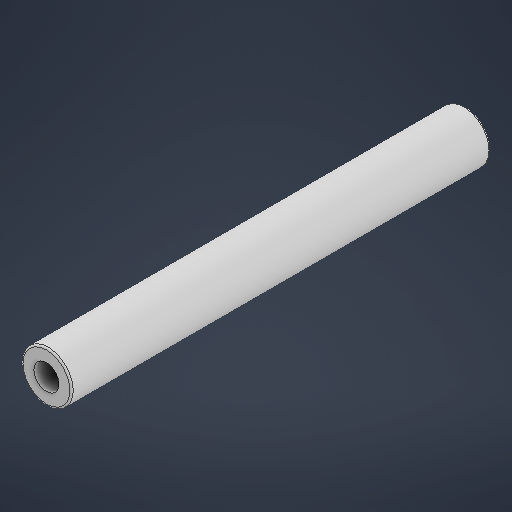
# Autodesk Inventor part: suport_bars
Saved by Autodesk Inventor 2025.3 (Build 293356000, 356)
## iProperties
Created: 2025-04-06
Part Number: suport_bars
Material: Generic
Document SubType Name: Modeling
Designer: Tiago
Density: 1 g/cm^3
Appearance: Default
Author: Tiago
Autodesk Inventor part; units mm, degrees
ref_plane "YZ Plane" through (0, 0, 0) normal (1, 0, 0) x (0, 1, 0)
ref_plane "XZ Plane" through (0, 0, 0) normal (0, 1, 0) x (-1, 0, 0)
ref_plane "XY Plane" through (0, 0, 0) normal (0, 0, 1) x (1, 0, 0)
sketch "Sketch1" plane through (0, 0, 0) normal (0, 0, 1) x (1, 0, 0)
  circle A0 centre (0, 0) radius 1.5
  circle A1 centre (0, 0) radius 3
  dimension "M3" = 3
  dimension "D" = 6
  constraints: 2 centre point, 2 coincident
  measures "M3" diameter of A0
  measures "D" diameter of A1
extrude "Extrusion3" add sketch "Sketch1" along normal blind 50
fillet "Fillet2" radius 0.2 2 edges at (-3, 0, 0) (-3, 0, 50)
body "Solid2"
